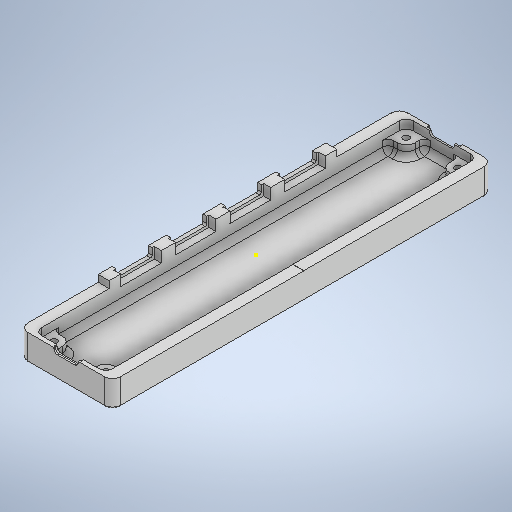
# Autodesk Inventor part: Lower_Housing
Saved by Autodesk Inventor 2025 (Build 290162010, 162A)
## iProperties
Created: 2025-09-30
Part Number: Lower_Housing
Material: Genérico
Document SubType Name: Modeling
Designer: João Vitor
Density: 1 g/cm^3
Appearance: Padrão
Author: João Vitor
Autodesk Inventor part; units mm, degrees
ref_plane "YZ Plane" through (0, 0, 0) normal (1, 0, 0) x (0, 1, 0)
ref_plane "XZ Plane" through (0, 0, 0) normal (0, 1, 0) x (-1, 0, 0)
ref_plane "XY Plane" through (0, 0, 0) normal (0, 0, 1) x (1, 0, 0)
sketch "Esboço1" plane through (0, 0, 0) normal (0, 1, 0) x (-1, 0, 0)
  line L0 (-10, 68) -> (10, 68)
  line L1 (13, 65) -> (13, -65)
  line L2 (10, -68) -> (-10, -68)
  line L3 (-13, -65) -> (-13, 65)
  line L4 (-13, 68) -> (13, -68) construction
  line L5 (13, 68) -> (-13, -68) construction
  circle A0 centre (9.5, 64.5) radius 1.2
  circle A1 centre (-9.5, 64.5) radius 1.2
  circle A2 centre (-9.5, -64.5) radius 1.2
  circle A3 centre (9.5, -64.5) radius 1.2
  line L6 (-14, 69.5) -> (14, 69.5)
  line L7 (17, 66.5) -> (17, -66.5)
  line L8 (14, -69.5) -> (-14, -69.5)
  line L9 (-17, -66.5) -> (-17, 66.5)
  line L10 (-17, 69.5) -> (17, -69.5) construction
  line L11 (17, 69.5) -> (-17, -69.5) construction
  arc A4 (-14, 69.5) -> (-17, 66.5) centre (-14, 66.5) ccw
  arc A5 (-10, 68) -> (-13, 65) centre (-10, 65) ccw
  arc A6 (13, 65) -> (10, 68) centre (10, 65) ccw
  arc A7 (17, 66.5) -> (14, 69.5) centre (14, 66.5) ccw
  arc A8 (14, -69.5) -> (17, -66.5) centre (14, -66.5) ccw
  arc A9 (10, -68) -> (13, -65) centre (10, -65) ccw
  arc A10 (-13, -65) -> (-10, -68) centre (-10, -65) ccw
  arc A11 (-17, -66.5) -> (-14, -69.5) centre (-14, -66.5) ccw
  circle A12 centre (-9.5, 64.5) radius 3.2
  circle A13 centre (9.5, 64.5) radius 3.2
  circle A14 centre (9.5, -64.5) radius 3.2
  circle A15 centre (-9.5, -64.5) radius 3.2
  line L12 (-9.5, 61.3) -> (-13, 61.3)
  line L13 (-6.3, 64.5) -> (-6.3, 68)
  line L14 (6.3, 64.5) -> (6.3, 68)
  line L15 (9.5, 61.3) -> (13, 61.3)
  line L16 (-9.5, -61.3) -> (-13, -61.3)
  line L17 (-6.3, -64.5) -> (-6.3, -68)
  line L18 (6.3, -64.5) -> (6.3, -68)
  line L19 (9.5, -61.3) -> (13, -61.3)
  point P0 (0, 0)
  dimension "d0" = 136
  dimension "d1" = 26
  dimension "d2" = 3.5
  dimension "d3" = 3.5
  dimension "d4" = 3.5
  dimension "d5" = 3.5
  dimension "d6" = 2.4
  dimension "d7" = 4
  dimension "d8" = 1.5
  dimension "d9" = 3
  dimension "d12" = 2
  dimension "d13" = 2
  dimension "d14" = 2
  dimension "d15" = 2
  constraints: 40 end point, 26 point on line, 24 point on circle, 23 tangent, 16 centre point, 10 equal radius, 9 perpendicular, 4 coincident, 4 midpoint, 4 parallel, 2 horizontal, 2 horizontal alignment, 2 vertical alignment
  measures "d0" distance between parallel lines of L2 L0
  measures "d1" distance between parallel lines of L1 L3
  measures "d2" distance from line of L3 A1.centre
  measures "d3" distance from line of L0 A1.centre
  measures "d4" distance from line of L2 A3.centre
  measures "d5" distance from line of L1 A3.centre
  measures "d6" diameter of A2
  measures "d7" distance between parallel lines of L7 L1
  measures "d8" distance between parallel lines of L8 L2
  measures "d9" radius of A4
  measures "d12" radial gap between concentric circles of A12 A1
  measures "d13" radial gap between concentric circles of A13 A0
  measures "d14" radial gap between concentric circles of A15 A2
  measures "d15" radial gap between concentric circles of A14 A3
extrude "Extrusão1" add sketch "Esboço1" along normal blind 2.4 contours L0 L13 A12 L12 L3 A5 | L0 L14 A13 L15 L1 L19 A14 L18 L2 L17 A15 L16 L3 L12 A12 L13 | L0 A6 L1 L15 A13 L14 | A12 | A13 | L16 A15 L17 L2 A10 L3 | A15 | L1 A9 L2 L18 A14 L19 | A14 | A0 | A1 | A2 | A3
extrude "Extrusão2" add sketch "Esboço1" along normal blind 6.5 contours L0 L13 A12 L12 L3 A5 | L0 A6 L1 L15 A13 L14 | A12 | A13 | L16 A15 L17 L2 A10 L3 | A15 | L1 A9 L2 L18 A14 L19 | A14
extrude "Extrusão3" add sketch "Esboço1" along normal blind 6.5 contours L6 A7 L7 A8 L8 A11 L9 A4
fillet "Arredondamento1" radius 0.5 8 edges at (16.1213, 0, -68.6213) (0, 0, -69.5) (-16.1213, 0, -68.6213) (-17, 0, 0) (-16.1213, 0, 68.6213) (0, 0, 69.5) (16.1213, 0, 68.6213) (17, 0, 0)
fillet "Arredondamento2" radius 2 16 edges at (6.3, 2.4, -66.25) (11.25, 2.4, -61.3) (7.2373, 2.4, -62.2373) (0, 2.4, -68) (-7.2373, 2.4, -62.2373) (-6.3, 2.4, -66.25) (-11.25, 2.4, -61.3) (-13, 2.4, 0) (13, 2.4, 0) (11.25, 2.4, 61.3) (6.3, 2.4, 66.25) (7.2373, 2.4, 62.2373) (0, 2.4, 68) (-6.3, 2.4, 66.25) (-11.25, 2.4, 61.3) (-7.2373, 2.4, 62.2373)
fillet "Arredondamento3" radius 2 16 edges at (13, 5.45, 61.3) (12.4142, 2.9858, 60.7142) (6.3, 5.45, 68) (5.7142, 2.9858, 67.4142) (-12.4142, 2.9858, 60.7142) (-13, 5.45, 61.3) (-6.3, 5.45, 68) (-5.7142, 2.9858, 67.4142) (-12.4142, 2.9858, -60.7142) (-13, 5.45, -61.3) (-6.3, 5.45, -68) (-5.7142, 2.9858, -67.4142) (13, 5.45, -61.3) (12.4142, 2.9858, -60.7142) (6.3, 5.45, -68) (5.7142, 2.9858, -67.4142)
sketch "Esboço2" plane through (0, 6.5, 0) normal (0, 1, 0) x (1, 0, 0)
  point P0 (0, 0)
sketch "Esboço3" plane through (0, 6.5, 0) normal (0, 1, 0) x (1, 0, 0)
  arc A0 (6.3, 66) -> (4.3, 68) centre (4.3, 66) ccw projected
  line L0 (4.3, 68) -> (13, 68)
  line L1 (13, 68) -> (13, 59.3)
  line L2 (13, 59.3) -> (13, -68)
  arc A1 (4.3, -68) -> (6.3, -66) centre (4.3, -66) ccw projected
  line L3 (13, -68) -> (4.3, -68)
  line L4 (4.3, -68) -> (-13, -68)
  line L5 (4.3, -68) -> (-4.3, -68) projected
  line L6 (-13, -59.3) -> (-13, 59.3) projected
  line L7 (-13, -68) -> (-13, -59.3)
  line L8 (-13, -59.3) -> (-13, 68)
  arc A2 (-4.3, 68) -> (-6.3, 66) centre (-4.3, 66) ccw projected
  line L9 (-13, 68) -> (-4.3, 68)
  line L10 (-4.3, 68) -> (4.3, 68)
  line L11 (17, -66.5) -> (17, 66.5) projected
  arc A3 (17, 66.5) -> (14, 69.5) centre (14, 66.5) ccw projected
  line L12 (14, 69.5) -> (-14, 69.5) projected
  line L13 (-17, 66.5) -> (-17, -66.5) projected
  arc A4 (-14, 69.5) -> (-17, 66.5) centre (-14, 66.5) ccw projected
  arc A5 (-17, -66.5) -> (-14, -69.5) centre (-14, -66.5) ccw projected
  line L14 (-14, -69.5) -> (14, -69.5) projected
  arc A6 (14, -69.5) -> (17, -66.5) centre (14, -66.5) ccw projected
  point P0 (0, 0)
  constraints: 18 end point, 3 perpendicular, 3 tangent, 2 collinear, 1 horizontal, 1 point on circle, 1 point on line, 1 vertical
extrude "Extrusão5" add sketch "Esboço3" along normal blind 5.554
sketch "Esboço4" plane through (-17, 0.5, -66.5) normal (-1, 0, 0) x (0, 0, 1)
  line L0 (0, 11.554) -> (133, 11.554) projected
  line L1 (28.92, 11.554) -> (42.22, 11.554)
  line L2 (42.22, 11.554) -> (42.22, 9.194)
  line L3 (41.62, 8.594) -> (29.52, 8.594)
  line L4 (28.92, 9.194) -> (28.92, 11.554)
  line L5 (48.92, 11.554) -> (62.22, 11.554)
  line L6 (62.22, 11.554) -> (62.22, 9.194)
  line L7 (61.62, 8.594) -> (49.52, 8.594)
  line L8 (48.92, 9.194) -> (48.92, 11.554)
  line L9 (68.92, 11.554) -> (82.22, 11.554)
  line L10 (82.22, 11.554) -> (82.22, 9.194)
  line L11 (81.62, 8.594) -> (69.52, 8.594)
  line L12 (68.92, 9.194) -> (68.92, 11.554)
  line L13 (88.92, 11.554) -> (102.22, 11.554)
  line L14 (102.22, 11.554) -> (102.22, 9.194)
  line L15 (101.62, 8.594) -> (89.52, 8.594)
  line L16 (88.92, 9.194) -> (88.92, 11.554)
  line L17 (-3, 0) -> (-3, 11.554) projected
  arc A0 (28.92, 9.194) -> (29.52, 8.594) centre (29.52, 9.194) ccw
  arc A1 (41.62, 8.594) -> (42.22, 9.194) centre (41.62, 9.194) ccw
  arc A2 (48.92, 9.194) -> (49.52, 8.594) centre (49.52, 9.194) ccw
  arc A3 (68.92, 9.194) -> (69.52, 8.594) centre (69.52, 9.194) ccw
  arc A4 (81.62, 8.594) -> (82.22, 9.194) centre (81.62, 9.194) ccw
  arc A5 (88.92, 9.194) -> (89.52, 8.594) centre (89.52, 9.194) ccw
  arc A6 (61.62, 8.594) -> (62.22, 9.194) centre (61.62, 9.194) ccw
  arc A7 (101.62, 8.594) -> (102.22, 9.194) centre (101.62, 9.194) ccw
  point P0 (66.5, -0.5)
  point P1 (28.92, 8.594)
  point P2 (62.22, 8.594)
  point P3 (82.22, 8.594)
  point P4 (102.22, 8.594)
  point P5 (28.92, 10.374)
  point P6 (48.92, 10.374)
  point P7 (68.92, 10.374)
  point P8 (62.22, 10.374)
  point P9 (88.92, 10.374)
  point P10 (82.22, 10.374)
  dimension "d27" = 13.3
  dimension "d28" = 31.92
  dimension "d29" = 6.7
  dimension "d32" = 2.96
  dimension "d33" = 0.6
  dimension "d34" = 6.7
  dimension "d35" = 0.6
  dimension "d36" = 6.7
  dimension "d37" = 0.6
  dimension "d38" = 0.6
  constraints: 32 end point, 16 point on circle, 16 tangent, 15 point on line, 8 centre point, 8 parallel, 6 midpoint, 4 equal radius, 4 horizontal, 4 perpendicular, 3 collinear
  measures "d27" distance between parallel lines of L2 L4
  measures "d28" distance from line of L17 point (28.92, 10.374)
  measures "d29" distance from line of point (48.92, 10.374) L2
  measures "d32" distance of point (28.92, 8.594) L1.start
  measures "d33" radius of A0
  measures "d34" distance between parallel lines of L12 L6
  measures "d35" radius of A3
  measures "d36" distance between parallel lines of L16 L10
  measures "d37" radius of A5
  measures "d38" radius of A7
extrude "Extrusão6" cut sketch "Esboço4" against normal blind 1.4
sketch "Esboço5" plane through (0, 12.054, 0) normal (0, 1, 0) x (1, 0, 0)
  line L0 (-15.6, 37.58) -> (-15.6, 24.28) projected
  line L1 (-15.6, 37.58) -> (-15.6, 38.355)
  line L2 (-13, -68) -> (-13, 68) projected
  line L3 (-15.6, 38.355) -> (-13, 38.355)
  line L4 (-15.6, 24.28) -> (-17, 24.28) projected
  line L5 (-15.6, 24.28) -> (-15.6, 23.505)
  line L6 (-15.6, 23.505) -> (-13, 23.505)
  line L7 (-15.6, 17.58) -> (-15.6, 4.28) projected
  line L8 (-15.6, 17.58) -> (-15.6, 18.355)
  line L9 (-15.6, 18.355) -> (-13, 18.355)
  line L10 (-15.6, 4.28) -> (-15.6, 3.505)
  line L11 (-15.6, 3.505) -> (-13, 3.505)
  line L12 (-17, -2.42) -> (-15.6, -2.42) projected
  line L13 (-15.6, -2.42) -> (-15.6, -1.645)
  line L14 (-15.6, -1.645) -> (-13, -1.645)
  line L15 (-15.6, -15.72) -> (-17, -15.72) projected
  line L16 (-17, -22.42) -> (-15.6, -22.42) projected
  line L17 (-15.6, -35.72) -> (-17, -35.72) projected
  line L18 (-17, -15.72) -> (-15.6, -15.72) projected
  line L19 (-15.6, -15.72) -> (-15.6, -16.495)
  line L20 (-15.6, -16.495) -> (-13, -16.495)
  line L21 (-15.6, -22.42) -> (-15.6, -21.645)
  line L22 (-15.6, -21.645) -> (-13, -21.645)
  line L23 (-15.6, -35.72) -> (-15.6, -36.495)
  line L24 (-15.6, -36.495) -> (-13, -36.495)
  line L25 (-15.6, -2.42) -> (-15.6, -15.72) projected
  line L26 (-15.6, -22.42) -> (-15.6, -35.72) projected
  point P0 (0, 0)
  point P1 (-15.6, 30.93)
  dimension "d41" = 14.85
  dimension "d42" = 7.425
  constraints: 32 end point, 6 collinear, 6 horizontal, 4 point on line, 4 vertical, 2 perpendicular, 1 midpoint, 9 other
  measures "d41" distance between parallel lines of L6 L3
  measures "d42" distance from line of point (-15.6, 30.93) L3
extrude "Extrusão7" cut sketch "Esboço5" against normal blind 3.96
sketch "Esboço6" plane through (14, 0.5, -69.5) normal (0, 0, -1) x (-1, 0, 0)
  point P0 (14, -0.5)
sketch "Esboço7" plane through (14, 0.5, -69.5) normal (0, 0, -1) x (-1, 0, 0)
  line L0 (-3, 0) -> (-3, 11.554) projected
  line L1 (0, 11.554) -> (-3, 11.554) projected
  line L2 (0, 11.554) -> (28, 11.554) projected
  line L3 (31, 0) -> (31, 11.554) projected
  line L4 (31, 11.554) -> (28, 11.554) projected
  line L5 (28, 0) -> (28, 11.554) projected
  line L6 (30.5, -0.5) -> (28, -0.5) projected
  arc A0 (30.5, -0.5) -> (31, 0) centre (30.5, 0) ccw projected
  line L7 (28, 0) -> (0, 0) projected
  line L8 (0, -0.5) -> (28, -0.5) projected
  line L9 (0, -0.5) -> (-2.5, -0.5) projected
  arc A1 (-3, 0) -> (-2.5, -0.5) centre (-2.5, 0) ccw projected
  line L10 (0, 0) -> (0, 11.554) projected
  line L11 (-3, 0) -> (0, 0) projected
  line L12 (28, 0) -> (31, 0) projected
  line L13 (28, 0) -> (28, -0.5) projected
  line L14 (1, 6) -> (9.7, 6) projected
  line L15 (-3, 9.139) -> (31, 9.139)
  line L16 (9.43, 9.139) -> (9.43, 8.839)
  line L17 (10.81, 7.459) -> (17.19, 7.459)
  line L18 (18.57, 8.839) -> (18.57, 9.139)
  line L19 (1, 6) -> (1, 11.554) projected
  arc A2 (9.43, 8.839) -> (10.81, 7.459) centre (10.81, 8.839) ccw
  arc A3 (17.19, 7.459) -> (18.57, 8.839) centre (17.19, 8.839) ccw
  point P0 (14, -0.5)
  point P1 (9.43, 7.459)
  point P2 (18.57, 7.459)
  point P3 (9.43, 8.989)
  point P4 (1, 9.139)
  point P5 (28, 9.139)
  dimension "d45" = 3.139
  dimension "d47" = 9.14
  dimension "d48" = 8.43
  dimension "d49" = 1.68
  dimension "d50" = 1.38
  constraints: 8 end point, 8 point on line, 4 point on circle, 4 tangent, 2 centre point, 2 horizontal, 1 equal radius, 1 midpoint, 1 perpendicular, 1 vertical
  measures "d45" distance between parallel lines of L15 L14
  measures "d47" distance of point (9.43, 7.459) point (18.57, 7.459)
  measures "d48" distance between parallel lines of L16 L19
  measures "d49" distance of L16.start point (9.43, 7.459)
  measures "d50" radius of A2
extrude "Extrusão8" cut sketch "Esboço7" against normal up to surface (1.5 mm away) contours L19 L2 L5 L15 | L15 L18 A3 L17 A2 L16
sketch "Esboço8" plane through (14, 0.5, -69.5) normal (0, 0, -1) x (-1, 0, 0)
  line L0 (9.43, 9.139) -> (1, 9.139) projected
  line L1 (7.93, 9.139) -> (7.93, 8.839)
  line L2 (10.81, 5.959) -> (17.19, 5.959)
  line L3 (20.07, 8.839) -> (20.07, 9.1431)
  line L4 (17.19, 7.459) -> (10.81, 7.459) projected
  line L5 (18.57, 9.139) -> (18.57, 8.839) projected
  line L6 (9.43, 8.839) -> (9.43, 9.139) projected
  arc A0 (7.93, 8.839) -> (10.81, 5.959) centre (10.81, 8.839) ccw
  arc A1 (17.19, 5.959) -> (20.07, 8.839) centre (17.19, 8.839) ccw
  arc A2 (9.43, 8.839) -> (10.81, 7.459) centre (10.81, 8.839) ccw projected
  arc A3 (17.19, 7.459) -> (18.57, 8.839) centre (17.19, 8.839) ccw projected
  line L7 (28, 9.139) -> (18.57, 9.139) projected
  point P0 (14, -0.5)
  point P1 (20.07, 9.139)
  dimension "d53" = 1.5
  dimension "d54" = 1.5
  dimension "d55" = 1.5
  dimension "d56" = 2.88
  constraints: 6 end point, 4 point on circle, 4 tangent, 3 perpendicular, 2 centre point, 1 equal radius, 1 point on line
  measures "d53" distance between parallel lines of L4 L2
  measures "d54" distance between parallel lines of L3 L5
  measures "d55" distance between parallel lines of L6 L1
  measures "d56" radius of A0
extrude "Extrusão9" cut sketch "Esboço8" against normal blind 0.9
sketch "Esboço10" plane through (-14, 0.5, 69.5) normal (0, 0, 1) x (1, 0, 0)
  line L0 (0, 11.554) -> (28, 11.554) projected
  line L1 (0, -0.5) -> (28, -0.5) projected
  line L2 (-3, 0) -> (-3, 11.554) projected
  line L3 (31, 0) -> (31, 11.554) projected
  line L4 (1, 6) -> (9.7, 6) projected
  line L5 (1, 6) -> (1, 11.554) projected
  line L6 (28, 0) -> (28, 11.554) projected
  line L7 (1, 9.064) -> (28, 9.064)
  line L8 (9.53, 9.064) -> (18.47, 9.064)
  line L9 (18.47, 9.064) -> (18.47, 8.6287)
  line L10 (17.19, 7.3487) -> (10.81, 7.3487)
  line L11 (9.53, 8.6287) -> (9.53, 9.064)
  arc A0 (9.53, 8.6287) -> (10.81, 7.3487) centre (10.81, 8.6287) ccw
  arc A1 (17.19, 7.3487) -> (18.47, 8.6287) centre (17.19, 8.6287) ccw
  point P0 (14, -0.5)
  point P1 (1, 9.139)
  point P2 (18.47, 7.3487)
  point P3 (9.53, 7.3487)
  dimension "d59" = 3.064
  dimension "d60" = 8.53
  dimension "d61" = 1.7153
  dimension "d62" = 8.94
  dimension "d63" = 1.28
  constraints: 10 end point, 7 point on line, 4 point on circle, 4 tangent, 2 centre point, 2 horizontal, 2 parallel, 1 equal radius, 1 perpendicular
  measures "d59" distance between parallel lines of L4 L7
  measures "d60" distance between parallel lines of L5 L11
  measures "d61" distance of L8.end point (18.47, 7.349)
  measures "d62" distance of point (18.47, 7.349) point (9.53, 7.349)
  measures "d63" radius of A0
extrude "Extrusão10" cut sketch "Esboço10" against normal up to surface (1.5 mm away)
sketch "Esboço11" plane through (13, 6.5, 68) normal (0, 0, -1) x (-1, 0, 0)
  line L0 (8.53, 3.064) -> (0, 3.064) projected
  line L1 (26, 3.064) -> (17.47, 3.064) projected
  line L2 (17.47, 3.064) -> (17.47, 2.6287) projected
  line L3 (16.19, 1.3487) -> (9.81, 1.3487) projected
  line L4 (8.53, 2.6287) -> (8.53, 3.064) projected
  line L5 (-1, 3.064) -> (8.53, 3.064) projected
  line L6 (8.13, 3.064) -> (8.13, 2.6287)
  line L7 (9.81, 0.9487) -> (13.1523, 0.9487)
  line L8 (13.1523, 0.9487) -> (16.19, 0.9487)
  line L9 (17.87, 2.6287) -> (17.87, 3.064)
  arc A0 (8.13, 2.6287) -> (9.81, 0.9487) centre (9.81, 2.6287) ccw
  arc A1 (16.19, 0.9487) -> (17.87, 2.6287) centre (16.19, 2.6287) ccw
  arc A2 (8.53, 2.6287) -> (9.81, 1.3487) centre (9.81, 2.6287) ccw projected
  arc A3 (16.19, 1.3487) -> (17.47, 2.6287) centre (16.19, 2.6287) ccw projected
  point P0 (13, -6.5)
  point P1 (17.87, 0.9487)
  point P2 (8.53, 2.8464)
  point P3 (8.13, 3.064)
  dimension "d66" = 0.4
  dimension "d67" = 0.4
  dimension "d68" = 0.4
  dimension "d69" = 1.68
  constraints: 8 end point, 5 point on line, 4 point on circle, 4 tangent, 2 centre point, 2 perpendicular, 1 equal radius, 1 midpoint, 1 vertical
  measures "d66" distance between parallel lines of L2 L9
  measures "d67" distance between parallel lines of L3 L8
  measures "d68" distance from line of point (8.53, 2.846) L6
  measures "d69" radius of A0
extrude "Extrusão11" cut sketch "Esboço11" against normal blind 0.9
sketch "Esboço12" plane through (-17, 0.5, -66.5) normal (-1, 0, 0) x (0, 0, 1)
  line L0 (-3, 9.139) -> (-3, 11.554) projected
  line L1 (-3, 9.139) -> (23.92, 9.139)
  line L2 (23.92, 9.139) -> (23.92, 11.554)
  line L3 (133, 11.554) -> (0, 11.554) projected
  line L4 (28.92, 9.194) -> (28.92, 11.554) projected
  line L5 (0, 11.554) -> (-3, 11.554) projected
  line L6 (134.5, 9.064) -> (135.4, 9.064) projected
  line L7 (136, 9.064) -> (134.5, 9.064) projected
  line L8 (136, 9.064) -> (107.22, 9.064)
  line L9 (107.22, 9.064) -> (107.22, 11.554)
  line L10 (102.22, 11.554) -> (102.22, 9.194) projected
  line L11 (136, 11.554) -> (133, 11.554) projected
  line L12 (136, 0) -> (136, 11.554) projected
  point P0 (66.5, -0.5)
  point P1 (-1.5, 9.139)
  point P2 (28.92, 10.374)
  point P3 (107.22, 10.309)
  dimension "d72" = 5
  dimension "d73" = 5
  constraints: 8 end point, 3 point on line, 2 midpoint, 2 perpendicular, 1 horizontal
  measures "d72" distance from line of point (28.92, 10.374) L2
  measures "d73" distance from line of point (107.22, 10.309) L10
extrude "Extrusão12" cut sketch "Esboço12" against normal up to surface (4 mm away)
sketch "Esboço13" plane through (17, 0.5, 66.5) normal (1, 0, 0) x (0, 0, -1)
  line L0 (-3.1481, 9.064) -> (136, 9.064)
  line L1 (133, 9.139) -> (136, 9.139) projected
  line L2 (136, 9.139) -> (-3, 9.139)
  line L3 (-3, 9.064) -> (-3, 11.554) projected
  line L4 (67, 9.139) -> (67, 9.064)
  line L5 (-3, 0) -> (-3, 9.064) projected
  line L6 (133, 0) -> (0, 0) projected
  line L7 (-3, 0) -> (0, 0) projected
  line L8 (0, 11.554) -> (133, 11.554) projected
  line L9 (0, 11.554) -> (-3, 11.554) projected
  line L10 (136, 11.554) -> (133, 11.554) projected
  line L11 (136, 0) -> (136, 11.554) projected
  point P0 (66.5, -0.5)
  point P1 (-1.5, 9.064)
  point P2 (134.5, 9.139)
  point P3 (-3, 9.0663)
  dimension "d79" = 70
  constraints: 6 end point, 4 point on line, 2 horizontal, 2 perpendicular, 1 parallel
  measures "d79" distance between parallel lines of L5 L4
fillet "Arredondamento4" radius 2.5 4 edges at (13, 8.0695, -68) (-13, 8.0695, -68) (13, 8.032, 68) (-13, 8.032, 68)
extrude "Extrusão14" cut sketch "Esboço13" against normal up to surface (4 mm away) contours L3 L2 L4 L0 | L3 L9 L8 L10 L11 L1 L2
equation "\"d10\" = d6"
